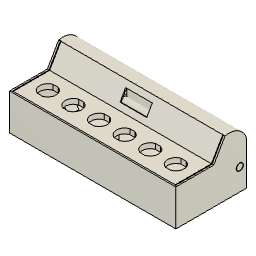
MiniMacro v14 (Autodesk Fusion 360 design; units mm, degrees)
Autodesk Fusion 360 part; units mm, degrees
note: some values were not read from the file. Set by a fixed rule: which sketch regions a step uses.
ref_plane "WorkPlane1" through (0, 35.5, 0) normal (0, 1, 0) x (0, 0, 1) in component "Top"
sketch "ButtonTop" plane through (0, 35.5, 0) normal (0, 1, 0) x (1, 0, 0) in component "Top"
  line L0 (-79, 17.75) -> (79, 17.75)
  line L1 (79, 17.75) -> (79, -17.75)
  line L2 (79, -17.75) -> (-79, -17.75)
  line L3 (-79, -17.75) -> (-79, 17.75)
  line L4 (-79, 17.75) -> (79, -17.75) construction
  line L5 (79, 17.75) -> (-79, -17.75) construction
  line L6 (-63, 17.75) -> (-63, -17.75) construction
  circle A0 centre (-63, 0) radius 8
  line L7 (-65.498, 7.6) -> (-60.502, 7.6)
  line L8 (-65.498, -7.6) -> (-60.502, -7.6)
  circle A1 centre (-38, 0) radius 8
  line L9 (-40.498, -7.6) -> (-35.502, -7.6)
  line L10 (-40.498, 7.6) -> (-35.502, 7.6)
  circle A2 centre (-13, 0) radius 8
  line L11 (-15.498, -7.6) -> (-10.502, -7.6)
  line L12 (-15.498, 7.6) -> (-10.502, 7.6)
  circle A3 centre (12, 0) radius 8
  line L13 (9.502, -7.6) -> (14.498, -7.6)
  line L14 (9.502, 7.6) -> (14.498, 7.6)
  circle A4 centre (37, 0) radius 8
  line L15 (34.502, -7.6) -> (39.498, -7.6)
  line L16 (34.502, 7.6) -> (39.498, 7.6)
  circle A5 centre (62, 0) radius 8
  line L17 (59.502, -7.6) -> (64.498, -7.6)
  line L18 (59.502, 7.6) -> (64.498, 7.6)
  dimension "d62" = 158
  dimension "d63" = 35.5
  dimension "d64" = 16
  dimension "d65" = 16
  dimension "d66" = 7.6
  dimension "d67" = 7.6
  dimension "d70" = 25
  dimension "d71" = 0
  constraint horizontal L0
  constraint perpendicular L0 L1
  constraint parallel L0 L2
  constraint parallel L1 L3
  constraint coincident L4 origin
  constraint coincident L5 origin
  constraint coincident L0 L6.start
  constraint coincident L2 L6.end
  constraint perpendicular L2 L6
  constraint midpoint L6 A0.centre
  constraint coincident A0 L7.start
  constraint coincident A0 L7.end
  constraint coincident A0 L8.start
  constraint coincident A0 L8.end
  constraint horizontal L7
  constraint horizontal L8
  measures "d62" distance of L1.end L2.end
  measures "d63" distance of L0.end L1.end
  measures "d64" distance of L3 L6
  measures "d65" diameter of A0
  measures "d66" distance of A0.centre L7
  measures "d67" distance of A0.centre L8
ref_plane "WorkPlane2" through (0, 35.5, -17.75) normal (0, 0.5, 0.866025) x (1, 0, 0) in component "Top"
sketch "DisplayTop" plane through (0, 1.189, 2.0595) normal (0, 0.5, 0.866025) x (1, 0, 0) in component "Top"
  line L0 (-79, 39.6189) -> (79, 39.6189)
  line L1 (-79, 39.6189) -> (-79, 61.6189)
  line L2 (79, 39.6189) -> (79, 61.6189)
  line L3 (-79, 61.6189) -> (79, 61.6189)
  line L4 (-79, 56.1189) -> (79, 56.1189) construction
  line L5 (-13, 56.1189) -> (13, 56.1189)
  line L6 (13, 56.1189) -> (13, 45.1189)
  line L7 (13, 45.1189) -> (-13, 45.1189)
  line L8 (-13, 45.1189) -> (-13, 56.1189)
  line L9 (0, 61.6189) -> (0, 39.6189) construction
  line L10 (-13, 44.3689) -> (13, 44.3689)
  line L11 (13, 44.3689) -> (13, 42.3689)
  line L12 (13, 42.3689) -> (-13, 42.3689)
  line L13 (-13, 42.3689) -> (-13, 44.3689)
  line L14 (-13, 58.8689) -> (13, 58.8689)
  line L15 (13, 58.8689) -> (13, 56.8689)
  line L16 (13, 56.8689) -> (-13, 56.8689)
  line L17 (-13, 56.8689) -> (-13, 58.8689)
  dimension "d73" = 22
  dimension "d74" = 22
  dimension "d75" = 5.5
  dimension "d76" = 26
  dimension "d77" = 11
  dimension "d78" = 13
  dimension "d183" = 26
  dimension "d184" = 2
  dimension "d185" = 0.75
  dimension "d186" = 26
  dimension "d187" = 2
  dimension "d188" = 0.75
  constraint coincident L0.start L1.start
  constraint perpendicular L0 L1
  constraint coincident L0.end L2.start
  constraint perpendicular L0 L2
  constraint coincident L1 L4.start
  constraint coincident L2 L4.end
  constraint perpendicular L2 L4
  constraint horizontal L5
  constraint vertical L6
  constraint horizontal L7
  constraint vertical L8
  constraint coincident L4 L5.start
  constraint midpoint L3 L9.start
  constraint midpoint L0 L9.end
  constraint horizontal L10
  constraint vertical L11
  constraint horizontal L12
  constraint vertical L13
  constraint collinear L8 L13
  constraint horizontal L14
  constraint vertical L15
  constraint horizontal L16
  constraint vertical L17
  constraint collinear L6 L15
  measures "d73" distance of L0.start L1.end
  measures "d74" distance of L0.end L2.end
  measures "d75" distance of L3 L4
  measures "d76" distance of L5.start L5.end
  measures "d77" distance of L5.start L7.end
  measures "d78" distance of L8 L9
  measures "d183" distance of L10.start L10.end
  measures "d184" distance of L10.start L12.end
  measures "d185" distance of L7 L10
  measures "d186" distance of L14.start L14.end
  measures "d187" distance of L14.start L16.end
  measures "d188" distance of L5 L16
extrude "Extrude1" add sketch "ButtonTop" against normal blind 5 contours L0 L1 L2 L3 | A0 L7 | A0 L8 | A1 L10 | A1 L9 | A2 L12 | A2 L11 | A3 L14 | A3 L13 | A4 L16 | A4 L15 | A5 L18 | A5 L17 makes body 1 in component "Top"
extrude "Extrude2" add sketch "DisplayTop" against normal blind 1.25 contours L0 L1 L2 L3 | L10 L11 L12 L13 | L14 L15 L16 L17 bodies 1 in component "Top"
sketch "SideProfile" plane through (79, 0, 0) normal (1, 0, 0) x (0, 0, -1) in component "Top"
  line L0 (17.75, 35.5) -> (-17.75, 35.5)
  line L1 (-17.75, 35.5) -> (-17.75, 30.5)
  line L2 (-17.75, 30.5) -> (17.75, 30.5)
  line L3 (17.75, 30.5) -> (17.75, 35.5)
  line L4 (28.75, 54.5526) -> (17.75, 35.5)
  line L5 (17.75, 35.5) -> (18.8325, 34.875)
  line L6 (18.8325, 34.875) -> (29.8325, 53.9276)
  line L7 (29.8325, 53.9276) -> (28.75, 54.5526)
  line L8 (18.8325, 34.875) -> (17.75, 30.5)
  constraint coincident L5.end L6.start
  constraint coincident L2.end L3.start
extrude "Extrude3" add sketch "SideProfile" against normal up to surface (158 mm away) contours L3 L5 L8 bodies 1 in component "Top"
sketch "Base" plane through (0, 0, 0) normal (0, 1, 0) x (1, 0, 0) in component "Walls"
  line L0 (-79.7, 0) -> (79.7, 0) construction
  line L1 (-79.7, -17.75) -> (79.7, -17.75)
  line L2 (-79.7, -17.75) -> (-79.7, 48.25)
  line L3 (79.7, -17.75) -> (79.7, 48.25)
  line L4 (-79.7, 48.25) -> (79.7, 48.25)
  line L5 (78.2, -16.25) -> (78.2, 46.75)
  line L6 (-78.2, 46.75) -> (78.2, 46.75)
  line L7 (-78.2, -16.25) -> (-78.2, 46.75)
  line L8 (-78.2, -16.25) -> (78.2, -16.25)
  line L9 (81.2, -19.25) -> (81.2, 49.75)
  line L10 (-81.2, 49.75) -> (81.2, 49.75)
  line L11 (-81.2, -19.25) -> (-81.2, 49.75)
  line L12 (-81.2, -19.25) -> (81.2, -19.25)
  line L13 (-81.2, 17.75) -> (81.2, 17.75)
  circle A0 centre (-71.7, -9.75) radius 8
  circle A1 centre (-71.7, 40.25) radius 8
  circle A2 centre (71.7, 40.25) radius 8
  circle A3 centre (71.7, -9.75) radius 8
  circle A4 centre (-71.7, -9.75) radius 2.25
  circle A5 centre (-71.7, 40.25) radius 2.25
  circle A6 centre (71.7, -9.75) radius 2.25
  circle A7 centre (71.7, 40.25) radius 2.25
  dimension "d86" = 159.4
  dimension "d87" = 66
  dimension "d88" = 17.75
  dimension "d93" = 1.5
  dimension "d94" = -1.5
  dimension "d99" = 17.75
  dimension "d114" = 8
  dimension "d115" = 8
  dimension "d116" = 8
  dimension "d117" = 8
  dimension "d118" = 4.5
  dimension "d119" = 4.5
  dimension "d120" = 4.5
  dimension "d121" = 4.5
  constraint horizontal L0
  constraint midpoint origin L0
  constraint horizontal L1
  constraint equal L0 L1
  constraint perpendicular L1 L2
  constraint perpendicular L1 L3
  constraint equal L2 L3
  constraint coincident L0.end L3
  constraint coincident L11 L13.start
  constraint coincident L9 L13.end
  constraint perpendicular L9 L13
  constraint tangent L2 A0
  constraint tangent L1 A0
  constraint tangent L2 A1
  constraint tangent L4 A1
  constraint tangent L4 A2
  constraint tangent L3 A2
  constraint tangent L3 A3
  constraint tangent L1 A3
  constraint concentric A0 A4
  constraint concentric A1 A5
  constraint concentric A3 A6
  constraint concentric A2 A7
  measures "d86" distance of L0.start L0.end
  measures "d87" distance of L1.start L2.end
  measures "d88" distance of L0 L1
  measures "d99" distance of L0 L13
  measures "d114" radius of A0
  measures "d115" radius of A1
  measures "d116" radius of A2
  measures "d117" radius of A3
  measures "d118" diameter of A4
  measures "d119" diameter of A5
  measures "d120" diameter of A6
  measures "d121" diameter of A7
extrude "Extrude2'" add sketch "Base" along normal blind 35.5 separate body contours L1 L2 L3 L9 L11 L12 L13 | L2 L3 L4 L9 L10 L11 L13 makes body 2 in component "Walls"
extrude "Extrude13" add sketch "Base" along normal blind 32.5 contours L1 L2 L7 L8 A0 | L1 L8 A0 A3 | L8 A0 | L2 L7 L13 A0 | L7 A0 | L1 L3 L5 L8 A3 | L8 A3 | L3 L5 L13 A3 | L5 A3 bodies 2 in component "Walls"
extrude "Extrude3'" add sketch "Base" along normal blind 24.5 contours L1 L2 L7 L8 A0 | L1 L8 A0 A3 | L8 A0 | L2 L7 L13 A0 | L7 A0 | L1 L3 L5 L8 A3 | L8 A3 | L7 L8 A0 | L7 L8 A0 | L5 L8 A3 | L5 L8 A3 | L2 L4 L6 L7 A1 | L7 A1 | L3 L5 L13 A3 | L5 A3 | L6 L7 A1 | L6 L7 A1 | L6 A1 | L5 L6 A2 | L5 A2 | L3 L4 L5 L6 A2 | L6 A2 | L5 L6 A2 | A4 | A5 | A6 | A7 bodies 2 in component "Walls"
extrude "Extrude5" add sketch "Base" along normal up to surface contours L2 L3 L4 L9 L10 L11 L13 | L2 L7 L13 A1 | L2 L4 L6 L7 A1 | L7 A1 | L3 L5 L13 A2 | L4 L6 A1 A2 | L6 A1 | L5 A2 | L3 L4 L5 L6 A2 | L6 A2 end surface through (-79, 54.5526, -28.75) normal (0, 0.866025, -0.5) offset 0 bodies 2 in component "Walls"
sketch "LSide" plane through (-81.2, 0, 0) normal (-1, 0, 0) x (0, 0, 1) in component "Walls"
  line L0 (-24.5, 45.7846) -> (-25.5825, 45.1596)
  line L1 (-49.75, 0) -> (19.25, 0)
  line L2 (19.25, 0) -> (19.25, 35.5)
  line L3 (19.25, 35.5) -> (-17.75, 35.5)
  line L4 (-17.75, 35.5) -> (-17.75, 60.9034)
  line L5 (-17.75, 60.9034) -> (-49.75, 42.4282)
  line L6 (-49.75, 42.4282) -> (-49.75, 0)
  line L7 (-17.75, 60.9034) -> (-49.75, 42.4282)
  line L8 (-17.75, 35.5) -> (-28.75, 54.5526)
  line L9 (-18.8325, 34.875) -> (-29.8325, 53.9276)
  line L10 (-17.75, 35.5) -> (-17.75, 60.9034)
  arc A0 (-28.75, 54.5526) -> (-49.75, 42.4282) centre (-32.7502, 37.2324) ccw
  line L11 (-17.75, 32.5) -> (-17.75, 35.5)
  line L12 (-17.75, 35.5) -> (17.75, 35.5)
  line L13 (17.75, 35.5) -> (17.75, 32.5)
  line L14 (17.75, 32.5) -> (-17.75, 32.5)
  line L15 (-18.8325, 34.875) -> (-17.75, 32.5)
  dimension "d132" = 17.7761
  constraint coincident L8.end A0.start
  constraint coincident L5.end L6.start
  constraint coincident L9.start L15.start
  constraint coincident L11.start L14.end
  measures "d132" radius of A0
extrude "Extrude6" cut sketch "LSide" along normal up to surface (0 mm away) and the other way up to surface (162.4 mm away) contours L4 L5 L7 L8 L10 bodies 2 in component "Walls"
extrude "Extrude7" add sketch "LSide" against normal blind 162.4 contours L5 L7 A0 bodies 2 in component "Walls"
extrude "Extrude8" cut sketch "Base" along normal blind 4 contours L1 L2 L7 L8 A0 | L1 L8 A0 A3 | L8 A0 | L2 L7 L13 A0 | L7 A0 | L1 L3 L5 L8 A3 | L8 A3 | L7 L8 A0 | L7 L8 A0 | L2 L7 L13 A1 | L5 L8 A3 | L5 L8 A3 | L2 L4 L6 L7 A1 | L7 A1 | L3 L5 L13 A3 | L5 A3 | L6 L7 A1 | L6 L7 A1 | L3 L5 L13 A2 | L4 L6 A1 A2 | L6 A1 | L5 L6 A2 | L5 A2 | L3 L4 L5 L6 A2 | L6 A2 | L5 L6 A2 | A4 | A5 | A6 | A7 bodies 2 in component "Walls"
sketch "Bottom" plane through (0, 0, 0) normal (0, 1, 0) x (1, 0, 0) in component "Bottom"
  circle A0 centre (-56.7, 43.25) radius 1.5
  line L0 (-56.7, 43.25) -> (-22.7, 43.25) construction
  line L1 (-22.7, 43.25) -> (-22.7, -13.75) construction
  line L2 (-22.7, -13.75) -> (-56.7, -13.75) construction
  line L3 (-56.7, -13.75) -> (-56.7, 43.25) construction
  circle A1 centre (-22.7, 43.25) radius 1.5
  circle A2 centre (-56.7, -13.75) radius 1.5
  circle A3 centre (-22.7, -13.75) radius 1.5
  line L4 (-22.7, 24.25) -> (-17.7, 24.25)
  line L5 (-17.7, 24.25) -> (-17.7, 14.25)
  line L6 (-17.7, 14.25) -> (-22.7, 14.25)
  line L7 (-22.7, 14.25) -> (-22.7, 24.25)
  line L8 (-19.7, 24.25) -> (-19.7, 14.25)
  line L9 (-61.7, 24.25) -> (-56.7, 24.25)
  line L10 (-56.7, 24.25) -> (-56.7, 14.25)
  line L11 (-56.7, 14.25) -> (-61.7, 14.25)
  line L12 (-61.7, 14.25) -> (-61.7, 24.25)
  line L13 (-59.7, 24.25) -> (-59.7, 14.25)
  circle A4 centre (-71.7, 40.25) radius 1.75
  circle A5 centre (-71.7, -9.75) radius 1.75
  circle A6 centre (71.7, 40.25) radius 1.75
  circle A7 centre (71.7, -9.75) radius 1.75
  circle A8 centre (-71.7, 40.25) radius 2.5
  circle A9 centre (-71.7, -9.75) radius 2.5
  circle A10 centre (71.7, 40.25) radius 2.5
  circle A11 centre (71.7, -9.75) radius 2.5
  line L14 (-81.2, 49.75) -> (81.2, 49.75)
  line L15 (-81.2, -19.25) -> (-81.2, 49.75)
  line L16 (-81.2, -19.25) -> (81.2, -19.25)
  line L17 (81.2, -19.25) -> (81.2, 49.75)
  line L18 (-81.2, 49.75) -> (81.2, 49.75)
  line L19 (-81.2, 49.75) -> (-81.2, 28.75)
  line L20 (-81.2, 17.75) -> (-81.2, 28.75)
  line L21 (-81.2, 17.75) -> (-81.2, -19.25)
  line L22 (-81.2, -19.25) -> (81.2, -19.25)
  line L23 (81.2, -19.25) -> (81.2, 17.75)
  line L24 (81.2, 28.75) -> (81.2, 17.75)
  line L25 (81.2, 28.75) -> (81.2, 49.75)
  line L26 (79.2, -17.75) -> (79.2, 48.25)
  line L27 (-79.7, 48.25) -> (79.2, 48.25)
  line L28 (-79.7, -17.75) -> (-79.7, 48.25)
  line L29 (-79.7, -17.75) -> (79.2, -17.75)
  point P0 (-71.7, 40.25)
  point P1 (-71.7, -9.75)
  point P2 (71.7, -9.75)
  point P3 (71.7, 40.25)
  dimension "d124" = 3
  dimension "d127" = 34
  dimension "d128" = 57
  dimension "d129" = 3
  dimension "d130" = 3
  dimension "d131" = 3
  dimension "d134" = 5
  dimension "d135" = 10
  dimension "d136" = 19
  dimension "d137" = 5
  dimension "d138" = 2
  dimension "d139" = 5
  dimension "d140" = 10
  dimension "d141" = 19
  dimension "d142" = 5
  dimension "d143" = 2
  dimension "d153" = 3.5
  dimension "d154" = 3.5
  dimension "d155" = 3.5
  dimension "d156" = 3.5
  dimension "d157" = 5
  dimension "d158" = 5
  dimension "d159" = 5
  dimension "d160" = 5
  dimension "d213" = 4
  dimension "d214" = 23
  constraint horizontal L0
  constraint vertical L1
  constraint horizontal L2
  constraint vertical L3
  constraint coincident A0.centre L0.start
  constraint coincident L0.end L1.start
  constraint coincident L2.end L3.start
  constraint coincident L1.end L2.start
  constraint horizontal L4
  constraint vertical L5
  constraint horizontal L6
  constraint vertical L7
  constraint coincident L4 L8.start
  constraint coincident L6 L8.end
  constraint perpendicular L6 L8
  constraint horizontal L9
  constraint vertical L10
  constraint horizontal L11
  constraint vertical L12
  constraint coincident L9 L13.start
  constraint coincident L11 L13.end
  constraint perpendicular L11 L13
  constraint coincident P0 A4.centre
  constraint coincident P1 A5.centre
  constraint coincident P3 A6.centre
  constraint coincident P2 A7.centre
  constraint concentric A4 A8
  measures "d124" diameter of A0
  measures "d127" distance of A0.centre L0.end
  measures "d128" distance of A0.centre L2.end
  measures "d129" diameter of A1
  measures "d130" diameter of A2
  measures "d131" diameter of A3
  measures "d134" distance of L4.start L4.end
  measures "d135" distance of L4.start L6.end
  measures "d136" distance of L0 L4
  measures "d137" distance of L1 L5
  measures "d138" distance of L5 L8
  measures "d139" distance of L9.start L9.end
  measures "d140" distance of L9.start L11.end
  measures "d141" distance of L0 L9
  measures "d142" distance of L3 L12
  measures "d143" distance of L12 L13
  measures "d153" diameter of A4
  measures "d154" diameter of A5
  measures "d155" diameter of A6
  measures "d156" diameter of A7
  measures "d157" diameter of A8
  measures "d158" diameter of A9
  measures "d159" diameter of A10
  measures "d160" diameter of A11
  measures "d213" distance of L1.end L29
  measures "d214" distance of A0.centre L28
extrude "Extrude1'" add sketch "Bottom" along normal blind 3 separate body contours A0 | A1 | A2 | A3 | L4 L6 L7 L8 | L4 L5 L6 L8 | L9 L11 L12 L13 | L9 L10 L11 L13 | A8 | A9 | A10 | A11 | L26 L27 L28 L29 makes body 3 in component "Bottom"
extrude "Extrude9" cut sketch "Base" along normal blind 11 contours A4 | A5 | A6 | A7 bodies 2 in component "Walls"
extrude "Extrude2''" add sketch "Bottom" along normal blind 8 contours A0 | A1 | A2 | A3 bodies 3 in component "Bottom"
extrude "Extrude3''" add sketch "Bottom" along normal blind 10.2 contours L4 L5 L6 L8 | L9 L11 L12 L13 bodies 3 in component "Bottom"
extrude "Extrude4" add sketch "Bottom" along normal blind 6 from surface at 10.2 contours L4 L6 L7 L8 | L4 L5 L6 L8 | L9 L11 L12 L13 | L9 L10 L11 L13 bodies 3 in component "Bottom"
sketch "ClipCutouts" plane through (0, 0, -14.25) normal (0, 0, 1) x (1, 0, 0) in component "Bottom"
  line L0 (-61.7, 3) -> (-59.7, 3)
  line L1 (-59.7, 3) -> (-59.7, 10.2)
  line L2 (-59.7, 10.2) -> (-56.7, 10.2)
  line L3 (-56.7, 10.2) -> (-56.7, 16.2)
  line L4 (-56.7, 16.2) -> (-61.7, 16.2)
  line L5 (-61.7, 16.2) -> (-61.7, 3)
  line L6 (-19.7, 3) -> (-17.7, 3)
  line L7 (-17.7, 3) -> (-17.7, 16.2)
  line L8 (-17.7, 16.2) -> (-22.7, 16.2)
  line L9 (-22.7, 16.2) -> (-22.7, 10.2)
  line L10 (-22.7, 10.2) -> (-19.7, 10.2)
  line L11 (-19.7, 10.2) -> (-19.7, 3)
  line L12 (-56.7, 10.2) -> (-61.7, 16.2)
  line L13 (-22.7, 10.2) -> (-17.7, 16.2)
  constraint coincident L2.end L3.start
  constraint coincident L4.end L5.start
  constraint coincident L7.end L8.start
  constraint coincident L9.end L10.start
extrude "Extrude5'" cut sketch "ClipCutouts" against normal up to surface (10 mm away) contours L3 L4 L12 | L8 L9 L13 bodies 3 in component "Bottom"
extrude "Extrude7'" cut sketch "Bottom" along normal blind 1.5 contours A8 | A9 | A10 | A11 bodies 3 in component "Bottom"
sketch "Back" plane through (0, 0, -49.75) normal (0, 0, -1) x (-1, 0, 0) in component "Walls"
  line L0 (-81.2, 0) -> (81.2, 0)
  line L1 (81.2, 0) -> (81.2, 42.4282)
  line L2 (81.2, 42.4282) -> (-81.2, 42.4282)
  line L3 (-81.2, 42.4282) -> (-81.2, 0)
  line L4 (22.7, 10.2) -> (17.7, 16.2)
  line L5 (17.7, 16.2) -> (17.7, 3)
  line L6 (17.7, 3) -> (19.7, 3)
  line L7 (19.7, 3) -> (19.7, 10.2)
  line L8 (19.7, 10.2) -> (22.7, 10.2)
  line L9 (61.7, 16.2) -> (56.7, 10.2)
  line L10 (56.7, 10.2) -> (59.7, 10.2)
  line L11 (59.7, 10.2) -> (59.7, 3)
  line L12 (59.7, 3) -> (61.7, 3)
  line L13 (61.7, 3) -> (61.7, 16.2)
  line L14 (32.7, 28.2) -> (47.7, 28.2)
  line L15 (47.7, 28.2) -> (47.7, 20.2)
  line L16 (47.7, 20.2) -> (32.7, 20.2)
  line L17 (32.7, 20.2) -> (32.7, 28.2)
  line L18 (-79.2, 0) -> (79.7, 0)
  line L19 (79.7, 0) -> (79.7, 3)
  line L20 (79.7, 3) -> (-79.2, 3)
  line L21 (-79.2, 3) -> (-79.2, 0)
  dimension "d170" = 15
  dimension "d171" = 8
  dimension "d172" = 17.2
  dimension "d173" = 12
  constraint horizontal L14
  constraint vertical L15
  constraint horizontal L16
  constraint vertical L17
  measures "d170" distance of L14.start L14.end
  measures "d171" distance of L14.start L16.end
  measures "d172" distance of L16 L20
  measures "d173" distance of L11 L15
extrude "Extrude10" cut sketch "Back" against normal up to surface (3 mm away) contours L14 L15 L16 L17 bodies 2 in component "Walls"
sketch "Sketch4" plane through (0, 1.189, 2.0595) normal (0, 0.5, 0.866025) x (1, 0, 0) in component "Walls"
  line L0 (-78.2, 39.6189) -> (-78.2, 61.6189)
  line L1 (-78.2, 61.6189) -> (-81.2, 61.6189)
  line L2 (-81.2, 61.6189) -> (-81.2, 39.6189)
  line L3 (-81.2, 39.6189) -> (-79.7, 39.6189)
  line L4 (-79.7, 39.6189) -> (-78.2, 39.6189)
  line L5 (81.2, 39.6189) -> (81.2, 61.6189)
  line L6 (81.2, 61.6189) -> (78.2, 61.6189)
  line L7 (78.2, 61.6189) -> (78.2, 39.6189)
  line L8 (78.2, 39.6189) -> (79.7, 39.6189)
  line L9 (79.7, 39.6189) -> (81.2, 39.6189)
  line L10 (79.6, 61.6189) -> (79.6, 39.6189)
  line L11 (-79.6, 61.6189) -> (-79.6, 39.6189)
  line L12 (-79.7, 39.6189) -> (-79.7, 37.0208)
  line L13 (-79.7, 37.0208) -> (-78.2, 37.0208)
  line L14 (-78.2, 37.0208) -> (-78.2, 39.6189)
  line L15 (79.7, 39.6189) -> (78.2, 39.6189)
  line L16 (78.2, 39.6189) -> (78.2, 37.0208)
  line L17 (78.2, 37.0208) -> (79.7, 37.0208)
  line L18 (79.7, 37.0208) -> (79.7, 39.6189)
  dimension "d179" = 1.4
  dimension "d180" = 1.4
  constraint coincident L6 L10.start
  constraint coincident L8 L10.end
  constraint perpendicular L8 L10
  constraint coincident L1 L11.start
  constraint perpendicular L1 L11
  constraint coincident L4 L11.end
  measures "d179" distance of L7 L10
  measures "d180" distance of L0 L11
extrude "Extrude11" cut sketch "Sketch4" against normal blind 1.3 contours L0 L1 L4 L11 | L4 L12 L13 L14 | L8 L15 L16 L17 L18 | L6 L7 L8 L10 L15 bodies 2 in component "Walls"
extrude "Extrude4'" add sketch "DisplayTop" against normal blind 4 contours L10 L11 L12 L13 | L14 L15 L16 L17 bodies 1 in component "Top"
sketch "RSide" plane through (81.2, 0, 0) normal (1, 0, 0) x (0, 0, -1) in component "Walls"
  line L0 (28.75, 54.5526) -> (17.75, 35.5)
  line L1 (17.75, 35.5) -> (-19.25, 35.5)
  line L2 (-19.25, 35.5) -> (-19.25, 0)
  line L3 (-19.25, 0) -> (49.75, 0)
  line L4 (49.75, 0) -> (49.75, 42.4282)
  arc A0 (49.75, 42.4282) -> (28.75, 54.5526) centre (32.7502, 37.2324) ccw
  circle A1 centre (43.25, 21.2) radius 3.5
  dimension "d192" = 7
  dimension "d193" = 21.2
  dimension "d196" = 6.5
  measures "d192" diameter of A1
  measures "d193" distance of L3 A1.centre
  measures "d196" distance of L4 A1.centre
extrude "Extrude12" cut sketch "RSide" against normal blind 115 contours A1 bodies 2 in component "Walls"
sketch "Sketch1" plane through (81.2, 0, 0) normal (1, 0, 0) x (0, 0, -1) in component "ResetButton"
  circle A0 centre (43.25, 21.2) radius 3.5
  line L0 (28.75, 54.5526) -> (17.75, 35.5)
  line L1 (17.75, 35.5) -> (-19.25, 35.5)
  line L2 (-19.25, 35.5) -> (-19.25, 0)
  line L3 (-19.25, 0) -> (49.75, 0)
  line L4 (49.75, 0) -> (49.75, 42.4282)
  arc A1 (49.75, 42.4282) -> (28.75, 54.5526) centre (32.7502, 37.2324) ccw
  circle A2 centre (43.25, 21.2) radius 3.5
  circle A3 centre (43.25, 21.2) radius 3.1
  dimension "d199" = 6.2
  constraint concentric A2 A3
  measures "d199" diameter of A3
extrude "Extrude1''" add sketch "Sketch1" against normal blind 113 separate body contours A3 makes body 4 in component "ResetButton"
ref_plane "WorkPlane1" through (-0.25, 1.5, -15.25) normal (1, 0, 0) x (0, 0, -1) in component "Bottom"
sketch "Sketch3" plane through (-0.25, 0, 0) normal (1, 0, 0) x (0, 0, -1) in component "Bottom"
  line L0 (48.25, 0) -> (-17.75, 0)
  line L1 (-17.75, 0) -> (-17.75, 3)
  line L2 (-17.75, 3) -> (48.25, 3)
  line L3 (48.25, 3) -> (48.25, 0)
  circle A0 centre (43.25, 21.2) radius 3.1
  line L4 (39.25, 3) -> (47.25, 3)
  line L5 (47.25, 3) -> (47.25, 23)
  line L6 (47.25, 23) -> (39.25, 23)
  line L7 (39.25, 23) -> (39.25, 3)
  circle A1 centre (43.25, 21.2) radius 3.5
  dimension "d202" = 20
  dimension "d203" = 1
  dimension "d204" = 8
  dimension "d205" = 7
  constraint horizontal L4
  constraint vertical L5
  constraint horizontal L6
  constraint vertical L7
  constraint coincident L2 L4.start
  constraint concentric A0 A1
  measures "d202" distance of L4.start L6.end
  measures "d203" distance of L3 L5
  measures "d204" distance of L5 L7
  measures "d205" diameter of A1
extrude "Extrude9'" [suppressed] in component "Bottom"
component "Top" placed x (1, 0, 0) y (0, 1, 0) z (0, 0, 1) at (0, 0, 0)
component "Walls" placed x (1, 0, 0) y (0, 1, 0) z (0, 0, 1) at (0, 0, 0)
component "Bottom" placed x (1, 0, 0) y (0, 1, 0) z (0, 0, 1) at (0, 0, 0)
component "ResetButton" placed x (1, 0, 0) y (0, 1, 0) z (0, 0, 1) at (0, 0, 0)
equation "ButtonDiameter = 16 mm"
equation "ButtonCuttoff = 7.6 mm"
equation "ButtonSpacing = ( ButtonDiameter / 2 ) + 1 mm"
equation "DisplayAngle = 30 deg"
equation "BaseWidth = ( ButtonDiameter + ButtonSpacing ) * 6 + ButtonSpacing"
equation "BaseLength = ButtonDiameter * 2"
equation "BaseHeight = 35.5 mm"
equation "WallThickness = 3 mm"
equation "TopThickness = 5 mm"
equation "DisplayBaseLength = DisplayHoleLength * 2"
equation "DisplayHoleWidth = 26.0 mm"
equation "DisplayHoleLength = 11.0 mm"
equation "ButtonHeight = 20 mm"
equation "DisplayThickness1 = 3.25 mm" comment "Depth at which holders should connect"
equation "DisplayThickness2 = 10 mm" comment "Longest point of connectors"
equation "BoardWidth = 40 mm"
equation "BoardLength = 60 mm"
equation "BoardThickness = 1.8 mm"
equation "DistanceBottomUSB = 14.2 mm" comment "Bottom of main board to bottom of USB"
equation "USBHeight = 8 mm"
equation "USBWidth = 15.0 mm"
equation "USBExtent = 4.0 mm"
equation "d61 = BaseHeight"
equation "d62 = BaseWidth - 1 mm"
equation "d63 = BaseHeight"
equation "d64 = ButtonDiameter"
equation "d65 = ButtonDiameter"
equation "d66 = ButtonCuttoff"
equation "d67 = ButtonCuttoff"
equation "d70 = ButtonDiameter + ButtonSpacing"
equation "d72 = -DisplayAngle"
equation "d73 = DisplayBaseLength"
equation "d74 = d73"
equation "d75 = DisplayHoleLength / 2"
equation "d76 = DisplayHoleWidth"
equation "d77 = DisplayHoleLength"
equation "d78 = DisplayHoleWidth / 2"
equation "d79 = -TopThickness"
equation "d81 = -DisplayWallThickness"
equation "DisplayWallThickness = 1.25 mm"
equation "d86 = BaseWidth + 0.4 mm"
equation "d87 = BaseHeight + 30.5 mm"
equation "d88 = BaseHeight / 2"
equation "d93 = WallThickness / 2"
equation "d94 = -( WallThickness / 2 )"
equation "d95 = BaseHeight"
equation "d97 = BaseHeight - TopThickness - 6 mm"
equation "d99 = BaseHeight / 2"
equation "d110 = WallThickness + 1 mm"
equation "d112 = WallThickness"
equation "d115 = d114"
equation "d116 = d114"
equation "d117 = d114"
equation "d118 = d119"
equation "d120 = d119"
equation "d121 = d119"
equation "d122 = WallThickness + 8 mm"
equation "d127 = BoardWidth - ( d124 * 2 )"
equation "d128 = BoardLength - d124"
equation "d129 = d124"
equation "d130 = d124"
equation "d131 = d124"
equation "BoardDistanceFromedge = 20 mm"
equation "d134 = d139"
equation "d135 = d140"
equation "d136 = d128 / 3"
equation "d137 = d142"
equation "d138 = d143"
equation "d141 = d128 / 3"
equation "d144 = WallThickness + 5 mm"
equation "d146 = BoardThickness + 0.4 mm + WallThickness + 5 mm"
equation "d148 = BoardThickness + 0.4 mm + WallThickness + 5 mm"
equation "d154 = d153"
equation "d155 = d153"
equation "d156 = d153"
equation "d158 = d157"
equation "d159 = d157"
equation "d160 = d157"
equation "d163 = WallThickness / 2"
equation "d170 = USBWidth"
equation "d171 = USBHeight"
equation "d172 = DistanceBottomUSB + 3.0 mm"
equation "d183 = DisplayHoleWidth"
equation "d186 = DisplayHoleWidth"
equation "d188 = d185"
equation "ResetButtonDiameter = 7 mm"
equation "d192 = ResetButtonDiameter"
equation "d193 = ResetButtonHeight + 4 mm"
equation "ResetButtonWidth = 115 mm"
equation "ResetButtonHeight = d172"
equation "d196 = 3 mm + ( ResetButtonDiameter / 2 )"
equation "d197 = -ResetButtonWidth"
equation "d199 = ResetButtonDiameter - 0.8 mm"
equation "d200 = -( ResetButtonWidth - 2 mm )"
equation "d202 = ButtonHeight"
equation "d204 = ResetButtonDiameter + 1.0 mm"
equation "d205 = ResetButtonDiameter"
equation "d208 = BaseHeight - WallThickness"
equation "d213 = USBExtent"
equation "d214 = BoardDistanceFromedge + d124"
named bodies: "MainWalls"
